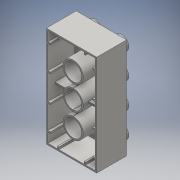
# Autodesk Inventor part: klarDupplo
Saved by Autodesk Inventor 2016 (Build 200138000, 138)
## iProperties
Created: 2017-02-13
Part Number: klarDupplo
Material: Generic
Document SubType Name: Modeling
Designer: 16wise
Density: 1 g/cm^3
Appearance: Default
Author: 16wise
Autodesk Inventor part; units mm, degrees
ref_plane "YZ Plane" through (0, 0, 0) normal (1, 0, 0) x (0, 1, 0)
ref_plane "XZ Plane" through (0, 0, 0) normal (0, 1, 0) x (-1, 0, 0)
ref_plane "XY Plane" through (0, 0, 0) normal (0, 0, 1) x (1, 0, 0)
sketch "Sketch1" plane through (0, 0, 0) normal (0, 1, 0) x (-1, 0, 0)
  line L0 (-16, 32) -> (16, 32)
  line L1 (16, 32) -> (16, -32)
  line L2 (16, -32) -> (-16, -32)
  line L3 (-16, -32) -> (-16, 32)
  line L4 (-16, 32) -> (16, -32) construction
  line L5 (16, 32) -> (-16, -32) construction
  point P0 (0, 0)
  dimension "d0" = 32
  dimension "d1" = 64
  constraints: 12 end point, 2 midpoint, 2 parallel, 1 horizontal, 1 perpendicular
  measures "d0" distance of L1.end L2.end
  measures "d1" distance of L0.end L1.end
extrude "Extrusion1" add sketch "Sketch1" along normal blind 19
sketch "Sketch2" plane through (0, 19, 0) normal (0, 1, 0) x (1, 0, 0)
  line L0 (-16, -32) -> (16, -32) projected
  line L1 (16, -32) -> (16, 32) projected
  line L2 (16, 32) -> (-16, 32) projected
  line L3 (-16, 32) -> (-16, -32) projected
  line L4 (-13, -29) -> (13, -29)
  line L5 (13, -29) -> (13, 29)
  line L6 (13, 29) -> (-13, 29)
  line L7 (-13, 29) -> (-13, -29)
  circle A0 centre (-8.5, -24.5) radius 4.5
  circle A1 centre (8.5, -24.5) radius 4.5
  line L8 (-16, 32) -> (-16, -32) projected
  circle A2 centre (-8.5, -8.2) radius 4.5
  circle A3 centre (-8.5, 8.1) radius 4.5
  circle A4 centre (-8.5, 24.4) radius 4.5
  circle A5 centre (8.5, -8.2) radius 4.5
  circle A6 centre (8.5, 8.1) radius 4.5
  circle A7 centre (8.5, 24.4) radius 4.5
  point P0 (0, 0)
  dimension "d4" = 3
  dimension "d5" = 9
  dimension "d6" = 9
  dimension "d9" = 16.3
  dimension "d16" = 16.3
  constraints: 8 centre point, 8 end point, 4 tangent, 2 vertical, 15 other
  measures "d4" distance between parallel lines of L3 L7
  measures "d5" diameter of A0
  measures "d6" diameter of A1
  measures "d9" distance of A0.centre A2.centre
  measures "d16" distance of A1.centre A5.centre
extrude "Extrusion2" add sketch "Sketch2" along normal blind 4.5 contours A5 | A6 | A7 | A4 | A3 | A2 | A0 | A1
sketch "Sketch3" plane through (-8.5, 23.5, 24.5) normal (0, 1, 0) x (1, 0, 0)
  circle A0 centre (0, 0) radius 3.5
  point P0 (8.5, 24.5)
  dimension "d23" = 7
  constraints: 1 centre point
  measures "d23" diameter of A0
extrude "Extrusion3" cut sketch "Sketch3" against normal blind 4.5
sketch "Sketch4" plane through (-8.5, 23.5, 8.2) normal (0, 1, 0) x (1, 0, 0)
  circle A0 centre (0, 0) radius 3.5
  point P0 (8.5, 8.2)
  dimension "d26" = 7
  constraints: 1 centre point
  measures "d26" diameter of A0
extrude "Extrusion4" cut sketch "Sketch4" against normal blind 4.5
sketch "Sketch5" plane through (-8.5, 23.5, -8.1) normal (0, 1, 0) x (1, 0, 0)
  circle A0 centre (0, 0) radius 3.5
  point P0 (8.5, -8.1)
  dimension "d29" = 7
  constraints: 1 centre point
  measures "d29" diameter of A0
extrude "Extrusion5" cut sketch "Sketch5" against normal blind 4.5
sketch "Sketch6" plane through (-8.5, 23.5, -24.4) normal (0, 1, 0) x (1, 0, 0)
  circle A0 centre (0, 0) radius 3.5
  point P0 (8.5, -24.4)
  dimension "d32" = 7
  constraints: 1 centre point
  measures "d32" diameter of A0
extrude "Extrusion6" cut sketch "Sketch6" against normal blind 4.5
sketch "Sketch7" plane through (8.5, 23.5, 24.5) normal (0, 1, 0) x (1, 0, 0)
  circle A0 centre (0, 0) radius 3.5
  point P0 (-8.5, 24.5)
  dimension "d35" = 7
  constraints: 1 centre point
  measures "d35" diameter of A0
extrude "Extrusion7" cut sketch "Sketch7" against normal blind 4.5
sketch "Sketch8" plane through (8.5, 23.5, 8.2) normal (0, 1, 0) x (1, 0, 0)
  circle A0 centre (0, 0) radius 4.5 projected
  circle A1 centre (0, 0) radius 3.5
  point P0 (-8.5, 8.2)
  dimension "d38" = 7
  constraints: 1 centre point, 1 coincident
  measures "d38" diameter of A1
extrude "Extrusion8" cut sketch "Sketch8" against normal blind 4.5 contours A1
sketch "Sketch9" plane through (8.5, 23.5, -8.1) normal (0, 1, 0) x (1, 0, 0)
  circle A0 centre (0, 0) radius 3.5
  point P0 (-8.5, -8.1)
  dimension "d41" = 7
  constraints: 1 centre point
  measures "d41" diameter of A0
extrude "Extrusion9" cut sketch "Sketch9" against normal blind 4.5
sketch "Sketch10" plane through (8.5, 23.5, -24.4) normal (0, 1, 0) x (1, 0, 0)
  circle A0 centre (0, 0) radius 3.5
  point P0 (-8.5, -24.4)
  dimension "d44" = 7
  constraints: 1 centre point
  measures "d44" diameter of A0
extrude "Extrusion10" cut sketch "Sketch10" against normal blind 4.5
sketch "Sketch11" plane through (0, 0, 0) normal (0, -1, 0) x (1, 0, 0)
  line L0 (16, 32) -> (-16, 32) projected
  line L1 (-16, 32) -> (-16, -32) projected
  line L2 (-16, -32) -> (16, -32) projected
  line L3 (16, -32) -> (16, 32) projected
  line L4 (15, -31) -> (-15, -31)
  line L5 (-15, -31) -> (-15, 31)
  line L6 (-15, 31) -> (15, 31)
  line L7 (15, 31) -> (15, -31)
  point P0 (0, 0)
  dimension "d47" = 1
  constraints: 8 end point, 3 other
  measures "d47" distance between parallel lines of L2 L4
extrude "Extrusion11" cut sketch "Sketch11" against normal blind 17 contours L4 L5 L6 L7
sketch "Sketch12" plane through (0, 17, 0) normal (0, -1, 0) x (1, 0, 0)
  circle A0 centre (0, 0) radius 6.5
  line L0 (15, -31) -> (-15, -31) projected
  line L1 (15, 31) -> (15, -31) projected
  line L2 (-15, 31) -> (15, 31) projected
  line L3 (-15, -31) -> (-15, 31) projected
  circle A1 centre (0, -15.5) radius 6.5
  circle A2 centre (0, 15.5) radius 6.5
  dimension "d50" = 13
  dimension "d53" = 15.5
  dimension "d60" = 15.5
  constraints: 3 centre point, 2 vertical, 1 coincident, 4 other
  measures "d50" diameter of A0
  measures "d53" distance of A0.centre A1.centre
  measures "d60" distance of A0.centre A2.centre
extrude "Extrusion12" add sketch "Sketch12" along normal blind 16 contours A0 | A1 | A2
sketch "Sketch13" plane through (0, 1, -15.5) normal (0, -1, 0) x (1, 0, 0)
  circle A0 centre (0, 0) radius 5.5
  circle A1 centre (0, 15.5) radius 5.5
  dimension "d67" = 11
  dimension "d68" = 11
  constraints: 2 centre point, 1 coincident
  measures "d67" diameter of A0
  measures "d68" diameter of A1
extrude "Extrusion13" cut sketch "Sketch13" against normal blind 16
sketch "Sketch14" plane through (0, 1, 15.5) normal (0, -1, 0) x (1, 0, 0)
  circle A0 centre (0, 0) radius 6.5 projected
  circle A1 centre (0, 0) radius 5.5
  point P0 (0, -15.5)
  dimension "d71" = 11
  constraints: 1 centre point, 1 coincident
  measures "d71" diameter of A1
extrude "Extrusion14" cut sketch "Sketch14" against normal blind 16 contours A1
sketch "Sketch15" plane through (0, 17, 0) normal (0, -1, 0) x (1, 0, 0)
  line L0 (-15, 0.5) -> (15, 0.5)
  line L1 (15, 0.5) -> (15, -0.5)
  line L2 (15, -0.5) -> (-15, -0.5)
  line L3 (-15, -0.5) -> (-15, 0.5)
  line L4 (-15, 0.5) -> (15, -0.5) construction
  line L5 (15, 0.5) -> (-15, -0.5) construction
  point P0 (0, 0)
  dimension "d74" = 30
  dimension "d75" = 1
  constraints: 12 end point, 2 midpoint, 2 parallel, 1 horizontal, 1 perpendicular
  measures "d74" distance of L1.end L2.end
  measures "d75" distance of L0.end L1.end
extrude "Extrusion15" add sketch "Sketch15" along normal blind 16
sketch "Sketch16" plane through (0, 1, 0) normal (0, -1, 0) x (1, 0, 0)
  arc A0 (5.4772, 0.5) -> (-5.4772, 0.5) centre (0, 0) ccw projected
  arc A1 (-5.4772, -0.5) -> (5.4772, -0.5) centre (0, 0) ccw projected
  line L0 (5.4772, 0.5) -> (5.4772, -0.5)
  line L1 (-5.4772, -0.5) -> (5.4772, -0.5) projected
  line L2 (-5.4772, 0.5) -> (-5.4772, -0.5)
  line L3 (-5.4772, -0.5) -> (5.4772, -0.5)
  line L4 (5.4772, 0.5) -> (-5.4772, 0.5) projected
  line L5 (5.4772, -0.5) -> (5.4772, 0.5)
  constraints: 8 end point, 2 vertical, 1 parallel, 1 perpendicular
extrude "Extrusion16" add sketch "Sketch16" against normal blind 16 contours L0 L1 L2 L4
sketch "Sketch17" plane through (0, 1, 0) normal (0, -1, 0) x (1, 0, 0)
  line L0 (5.4772, 0.5) -> (-5.4772, 0.5) projected
  line L1 (-5.4772, 0.5) -> (5.4772, 0.5)
  arc A0 (-5.4772, -0.5) -> (5.4772, -0.5) centre (0, 0) ccw projected
  arc A1 (5.4772, 0.5) -> (-5.4772, 0.5) centre (0, 0) ccw projected
  line L2 (5.4772, 0.5) -> (-5.4772, -0.5)
  line L3 (-5.4772, -0.5) -> (5.4772, -0.5) projected
  line L4 (-5.4772, -0.5) -> (-5.4772, 0.5)
  line L5 (5.4772, -0.5) -> (5.4772, 0.5)
  constraints: 8 end point, 2 equal length, 1 perpendicular
extrude "Extrusion17" cut sketch "Sketch17" against normal blind 16 contours L2 L4 L0 | L5 L3 L2
sketch "Sketch18" plane through (0, 17, 0) normal (0, -1, 0) x (1, 0, 0)
  circle A0 centre (0, 15.5) radius 6.5 projected
  line L0 (-0.25, -9.0048) -> (0.25, -9.0048)
  line L1 (0.25, -9.0048) -> (0.25, 9.0048)
  line L2 (0.25, 9.0048) -> (-0.25, 9.0048)
  line L3 (-0.25, 9.0048) -> (-0.25, -9.0048)
  line L4 (-0.25, -9.0048) -> (0.25, 9.0048) construction
  line L5 (0.25, -9.0048) -> (-0.25, 9.0048) construction
  point P0 (0, 0)
  dimension "d82" = 0.5
  constraints: 12 end point, 2 midpoint, 2 parallel, 1 horizontal, 1 perpendicular, 2 other
  measures "d82" distance of L2.end L1.end
extrude "Extrusion18" add sketch "Sketch18" along normal blind 16 contours L2 A0 | A0 L1 L0 L3 picked at (-0.0278, 9.0034)
sketch "Sketch19" plane through (0, 1, 0) normal (0, -1, 0) x (1, 0, 0)
  line L0 (0.25, 5.4943) -> (0.25, -5.4943) projected
  line L1 (-0.25, -5.4943) -> (0.25, -5.4943)
  line L2 (0.25, -5.4943) -> (0.25, 5.4943)
  line L3 (0.25, 5.4943) -> (-0.25, 5.4943)
  line L4 (-0.25, 5.4943) -> (-0.25, -5.4943)
  line L5 (-0.25, -5.4943) -> (0.25, 5.4943) construction
  line L6 (0.25, -5.4943) -> (-0.25, 5.4943) construction
  point P0 (0, 0)
  constraints: 12 end point, 2 midpoint, 2 parallel, 1 horizontal, 1 perpendicular
extrude "Extrusion19" cut sketch "Sketch19" against normal blind 16
sketch "Sketch20" plane through (0, 0, 0) normal (0, -1, 0) x (1, 0, 0)
  line L0 (15, -31) -> (-15, -31) projected
  line L1 (15, -31) -> (8, -31)
  line L2 (8, -31) -> (8, -24)
  line L3 (8, -24) -> (15, -24)
  line L4 (15, -24) -> (15, -31)
  point P0 (0, 0)
  dimension "d87" = 7
  dimension "d88" = 7
  constraints: 8 end point, 2 parallel, 1 horizontal, 1 perpendicular
  measures "d87" distance of L2.end L3.end
  measures "d88" distance of L1.end L2.end
extrude "Extrusion20" add sketch "Sketch20" against normal blind 16
sketch "Sketch21" plane through (0, 0, 0) normal (0, -1, 0) x (1, 0, 0)
  line L0 (15, -31) -> (-15, -31) projected
  line L1 (15, -31) -> (9, -31)
  line L2 (9, -31) -> (9, -25)
  line L3 (9, -25) -> (15, -25)
  line L4 (15, -25) -> (15, -31)
  point P0 (0, 0)
  dimension "d91" = 6
  dimension "d92" = 6
  constraints: 8 end point, 2 parallel, 1 horizontal, 1 perpendicular
  measures "d91" distance of L2.end L3.end
  measures "d92" distance of L1.end L2.end
extrude "Extrusion21" cut sketch "Sketch21" against normal blind 16
sketch "Sketch22" plane through (0, 1, 0) normal (0, -1, 0) x (1, 0, 0)
  line L0 (-0.25, 6.4952) -> (-0.25, 9.0048) projected
  line L1 (0.25, 9.0048) -> (0.25, 6.4952) projected
  line L2 (-0.25, 9.0048) -> (0.25, 9.0048)
  line L3 (0.25, 9.0048) -> (0.25, 6.4952)
  line L4 (0.25, 6.4952) -> (-0.25, 6.4952)
  line L5 (-0.25, 6.4952) -> (-0.25, 9.0048)
  point P0 (0, 0)
  constraints: 8 end point, 2 parallel, 1 horizontal, 1 perpendicular
extrude "Extrusion22" cut sketch "Sketch22" against normal blind 2.5
sketch "Sketch23" plane through (0, 1, 0) normal (0, -1, 0) x (1, 0, 0)
  arc A0 (-6.4807, -0.5) -> (-0.25, -6.4952) centre (0, 0) ccw projected
  arc A1 (-0.25, -9.0048) -> (0.25, -9.0048) centre (0, -15.5) ccw projected
  line L0 (-0.25, -6.4952) -> (0.25, -6.4952)
  line L1 (0.25, -6.4952) -> (0.25, -9.0048)
  line L2 (0.25, -9.0048) -> (-0.25, -9.0048)
  line L3 (-0.25, -9.0048) -> (-0.25, -6.4952)
  constraints: 8 end point, 2 parallel, 1 horizontal, 1 perpendicular
extrude "Extrusion23" cut sketch "Sketch23" against normal blind 2.5 contours L3 L0 L1 L2
sketch "Sketch24" plane through (0, 1, 0) normal (0, -1, 0) x (1, 0, 0)
  line L0 (-6.4807, 0.5) -> (-15, 0.5) projected
  line L1 (-15, -0.5) -> (-6.4807, -0.5) projected
  line L2 (-15, 0.5) -> (-6.4807, 0.5)
  line L3 (-6.4807, 0.5) -> (-6.4807, -0.5)
  line L4 (-6.4807, -0.5) -> (-15, -0.5)
  line L5 (-15, -0.5) -> (-15, 0.5)
  point P0 (0, 0)
  constraints: 8 end point, 2 parallel, 1 horizontal, 1 perpendicular
extrude "Extrusion24" cut sketch "Sketch24" against normal blind 3.5
sketch "Sketch25" plane through (0, 1, 0) normal (0, -1, 0) x (1, 0, 0)
  line L0 (15, 0.5) -> (6.4807, 0.5) projected
  line L1 (6.4807, -0.5) -> (15, -0.5) projected
  line L2 (6.4807, 0.5) -> (15, 0.5)
  line L3 (15, 0.5) -> (15, -0.5)
  line L4 (15, -0.5) -> (6.4807, -0.5)
  line L5 (6.4807, -0.5) -> (6.4807, 0.5)
  point P0 (0, 0)
  constraints: 8 end point, 2 parallel, 1 horizontal, 1 perpendicular
extrude "Extrusion25" cut sketch "Sketch25" against normal blind 3.5
sketch "Sketch26" plane through (0, 0, 0) normal (0, -1, 0) x (1, 0, 0)
  line L0 (-15, 31) -> (15, 31) projected
  line L1 (15, 31) -> (8, 31)
  line L2 (8, 31) -> (8, 24)
  line L3 (8, 24) -> (15, 24)
  line L4 (15, 24) -> (15, 31)
  point P0 (0, 0)
  dimension "d103" = 7
  dimension "d104" = 7
  constraints: 8 end point, 2 parallel, 1 horizontal, 1 perpendicular
  measures "d103" distance of L3.end L2.end
  measures "d104" distance of L2.end L1.end
extrude "Extrusion26" add sketch "Sketch26" against normal blind 18
sketch "Sketch27" plane through (0, 0, 0) normal (0, -1, 0) x (1, 0, 0)
  line L0 (-15, 0.5) -> (-15, 31) projected
  line L1 (-15, 31) -> (-8, 31)
  line L2 (-8, 31) -> (-8, 24)
  line L3 (-8, 24) -> (-15, 24)
  line L4 (-15, 24) -> (-15, 31)
  point P0 (0, 0)
  dimension "d107" = 7
  dimension "d108" = 7
  constraints: 8 end point, 2 parallel, 1 horizontal, 1 perpendicular
  measures "d107" distance of L2.end L3.end
  measures "d108" distance of L1.end L2.end
extrude "Extrusion27" add sketch "Sketch27" against normal blind 18
sketch "Sketch28" plane through (0, 0, 0) normal (0, -1, 0) x (1, 0, 0)
  line L0 (-15, -31) -> (-15, -0.5) projected
  line L1 (-15, -31) -> (-8, -31)
  line L2 (-8, -31) -> (-8, -24)
  line L3 (-8, -24) -> (-15, -24)
  line L4 (-15, -24) -> (-15, -31)
  point P0 (0, 0)
  dimension "d111" = 7
  dimension "d112" = 7
  constraints: 8 end point, 2 parallel, 1 horizontal, 1 perpendicular
  measures "d111" distance of L3.end L2.end
  measures "d112" distance of L2.end L1.end
extrude "Extrusion28" add sketch "Sketch28" against normal blind 18
sketch "Sketch29" plane through (0, 0, 0) normal (0, -1, 0) x (1, 0, 0)
  line L0 (15, 31) -> (9, 31)
  line L1 (9, 31) -> (9, 25)
  line L2 (9, 25) -> (15, 25)
  line L3 (15, 25) -> (15, 31)
  line L4 (-15, 31) -> (-9, 31)
  line L5 (-9, 31) -> (-9, 25)
  line L6 (-9, 25) -> (-15, 25)
  line L7 (-15, 25) -> (-15, 31)
  line L8 (-15, -31) -> (-9, -31)
  line L9 (-9, -31) -> (-9, -25)
  line L10 (-9, -25) -> (-15, -25)
  line L11 (-15, -25) -> (-15, -31)
  point P0 (0, 0)
  dimension "d115" = 6
  dimension "d116" = 6
  dimension "d117" = 6
  dimension "d118" = 6
  dimension "d119" = 6
  constraints: 24 end point, 6 parallel, 3 horizontal, 3 perpendicular, 3 point on line
  measures "d115" distance of L2.end L1.end
  measures "d116" distance of L1.end L0.end
  measures "d117" distance of L5.end L6.end
  measures "d118" distance of L10.end L9.end
  measures "d119" distance of L9.end L8.end
extrude "Extrusion29" cut sketch "Sketch29" against normal blind 18
sketch "Sketch30" plane through (0, 0, 0) normal (0, -1, 0) x (1, 0, 0)
  line L0 (-8, -24) -> (-15, -24) projected
  line L1 (-15, -25) -> (-9, -25) projected
  line L2 (-8, -24) -> (-13.5, -24)
  line L3 (-13.5, -24) -> (-13.5, -25)
  line L4 (-13.5, -25) -> (-8, -25)
  line L5 (-8, -25) -> (-8, -24)
  point P0 (0, 0)
  dimension "d122" = 5.5
  constraints: 8 end point, 2 parallel, 1 horizontal, 1 perpendicular, 1 point on line
  measures "d122" distance of L4.end L3.end
extrude "Extrusion30" cut sketch "Sketch30" against normal blind 17
sketch "Sketch31" plane through (0, 0, 0) normal (0, -1, 0) x (1, 0, 0)
  line L0 (-9, -25) -> (-13.5, -25) projected
  line L1 (-9, -25) -> (-8, -25)
  line L2 (-8, -25) -> (-8, -29.5)
  line L3 (-8, -29.5) -> (-9, -29.5)
  line L4 (-9, -29.5) -> (-9, -25)
  point P0 (0, 0)
  dimension "d125" = 1
  dimension "d126" = 4.5
  constraints: 8 end point, 2 parallel, 1 horizontal, 1 perpendicular
  measures "d125" distance of L2.end L3.end
  measures "d126" distance of L1.end L2.end
extrude "Extrusion31" cut sketch "Sketch31" against normal blind 17
sketch "Sketch32" plane through (0, 0, 0) normal (0, -1, 0) x (1, 0, 0)
  line L0 (8, -24) -> (15, -24) projected
  line L1 (9, -25) -> (15, -25) projected
  line L2 (8, -24) -> (13.5, -24)
  line L3 (13.5, -24) -> (13.5, -25)
  line L4 (13.5, -25) -> (8, -25)
  line L5 (8, -25) -> (8, -24)
  point P0 (0, 0)
  dimension "d129" = 5.5
  constraints: 8 end point, 2 parallel, 1 horizontal, 1 perpendicular, 1 point on line
  measures "d129" distance of L3.end L4.end
extrude "Extrusion32" cut sketch "Sketch32" against normal blind 17
sketch "Sketch33" plane through (0, 0, 0) normal (0, -1, 0) x (1, 0, 0)
  line L0 (8, -25) -> (9, -25)
  line L1 (9, -25) -> (9, -29.5)
  line L2 (9, -29.5) -> (8, -29.5)
  line L3 (8, -29.5) -> (8, -25)
  point P0 (0, 0)
  dimension "d132" = 1
  dimension "d133" = 4.5
  constraints: 8 end point, 2 parallel, 1 horizontal, 1 perpendicular
  measures "d132" distance of L1.end L2.end
  measures "d133" distance of L0.end L1.end
extrude "Extrusion33" cut sketch "Sketch33" against normal blind 17
sketch "Sketch34" plane through (0, 0, 0) normal (0, -1, 0) x (1, 0, 0)
  line L0 (8, 24) -> (15, 24) projected
  line L1 (8, 24) -> (9, 24)
  line L2 (9, 24) -> (9, 29.5)
  line L3 (9, 29.5) -> (8, 29.5)
  line L4 (8, 29.5) -> (8, 24)
  point P0 (0, 0)
  dimension "d136" = 1
  dimension "d137" = 5.5
  constraints: 8 end point, 2 parallel, 1 horizontal, 1 perpendicular
  measures "d136" distance of L3.end L2.end
  measures "d137" distance of L2.end L1.end
extrude "Extrusion34" cut sketch "Sketch34" against normal blind 17
sketch "Sketch35" plane through (0, 0, 0) normal (0, -1, 0) x (1, 0, 0)
  line L0 (15, 25) -> (9, 25) projected
  line L1 (15, 24) -> (9, 24) projected
  line L2 (9, 25) -> (13.5, 25)
  line L3 (13.5, 25) -> (13.5, 24)
  line L4 (13.5, 24) -> (9, 24)
  line L5 (9, 24) -> (9, 25)
  point P0 (0, 0)
  dimension "d140" = 4.5
  constraints: 8 end point, 2 parallel, 1 horizontal, 1 perpendicular, 1 point on line
  measures "d140" distance of L3.end L4.end
extrude "Extrusion35" cut sketch "Sketch35" against normal blind 17
sketch "Sketch36" plane through (0, 0, 0) normal (0, -1, 0) x (1, 0, 0)
  line L0 (-8, 31) -> (-8, 24) projected
  line L1 (-8, 24) -> (-9, 24)
  line L2 (-9, 24) -> (-9, 29.5)
  line L3 (-9, 29.5) -> (-8, 29.5)
  line L4 (-8, 29.5) -> (-8, 24)
  point P0 (0, 0)
  dimension "d143" = 1
  dimension "d144" = 5.5
  constraints: 8 end point, 2 parallel, 1 horizontal, 1 perpendicular
  measures "d143" distance of L2.end L3.end
  measures "d144" distance of L1.end L2.end
extrude "Extrusion36" cut sketch "Sketch36" against normal blind 17
sketch "Sketch37" plane through (0, 0, 0) normal (0, -1, 0) x (1, 0, 0)
  line L0 (-9, 25) -> (-9, 29.5) projected
  line L1 (-9, 24) -> (-15, 24) projected
  line L2 (-9, 25) -> (-13.5, 25)
  line L3 (-13.5, 25) -> (-13.5, 24)
  line L4 (-13.5, 24) -> (-9, 24)
  line L5 (-9, 24) -> (-9, 25)
  point P0 (0, 0)
  dimension "d147" = 4.5
  constraints: 8 end point, 2 parallel, 1 horizontal, 1 perpendicular, 1 point on line
  measures "d147" distance of L4.end L3.end
extrude "Extrusion37" cut sketch "Sketch37" against normal blind 17
sketch "Sketch40" plane through (0, 18, 0) normal (0, -1, 0) x (1, 0, 0)
  line L0 (-9, 31) -> (-9, 25) projected
  line L1 (-15, 31) -> (-9, 31) projected
  line L2 (-9, 25) -> (-15, 25)
  line L3 (-15, 25) -> (-15, 31)
  line L4 (-15, 31) -> (-9, 31)
  line L5 (-9, 31) -> (-9, 25)
  point P0 (0, 0)
  constraints: 8 end point, 2 parallel, 1 horizontal, 1 perpendicular
extrude "Extrusion38" add sketch "Sketch40" along normal blind 1
sketch "Sketch41" plane through (0, 18, 0) normal (0, -1, 0) x (1, 0, 0)
  line L0 (9, 29.5) -> (9, 25) projected
  line L1 (9, 31) -> (15, 31) projected
  line L2 (9, 25) -> (15, 25)
  line L3 (15, 25) -> (15, 31)
  line L4 (15, 31) -> (9, 31)
  line L5 (9, 31) -> (9, 25)
  point P0 (0, 0)
  constraints: 8 end point, 2 parallel, 1 horizontal, 1 perpendicular
extrude "Extrusion39" add sketch "Sketch41" along normal blind 1
sketch "Sketch42" plane through (0, 18, 0) normal (0, -1, 0) x (1, 0, 0)
  line L0 (-15, -25) -> (-9, -25) projected
  line L1 (-15, -31) -> (-15, -25) projected
  line L2 (-9, -25) -> (-15, -25)
  line L3 (-15, -25) -> (-15, -31)
  line L4 (-15, -31) -> (-9, -31)
  line L5 (-9, -31) -> (-9, -25)
  point P0 (0, 0)
  constraints: 8 end point, 2 parallel, 1 horizontal, 1 perpendicular
extrude "Extrusion40" add sketch "Sketch42" along normal blind 1
sketch "Sketch43" plane through (0, 1, 0) normal (0, -1, 0) x (1, 0, 0)
  line L0 (9, 31) -> (15, 31) projected
  line L1 (15, 31) -> (15, 8)
  line L2 (15, 24) -> (15, 0.5) projected
  line L3 (15, 8) -> (13.5, 8)
  line L4 (13.5, 8) -> (13.5, 7)
  line L5 (13.5, 7) -> (15, 7)
  line L6 (15, 7) -> (15, 8)
  line L7 (-15, 31) -> (-9, 31) projected
  line L8 (-15, 31) -> (-15, 9)
  line L9 (-15, 0.5) -> (-15, 24) projected
  line L10 (-15, 9) -> (-13.5, 9)
  line L11 (-13.5, 9) -> (-13.5, 8)
  line L12 (-13.5, 8) -> (-15, 8)
  line L13 (-15, 8) -> (-15, 9)
  line L14 (15, -0.5) -> (15, -31) projected
  line L15 (15, -31) -> (15, -9)
  line L16 (15, -9) -> (13.5, -9)
  line L17 (13.5, -9) -> (13.5, -8)
  line L18 (13.5, -8) -> (15, -8)
  line L19 (15, -8) -> (15, -9)
  line L20 (-15, -31) -> (-15, -25) projected
  line L21 (-15, -31) -> (-15, -9)
  line L22 (-15, -24) -> (-15, -0.5) projected
  line L23 (-15, -9) -> (-13.5, -9)
  line L24 (-13.5, -9) -> (-13.5, -8)
  line L25 (-13.5, -8) -> (-15, -8)
  line L26 (-15, -8) -> (-15, -9)
  point P0 (0, 0)
  dimension "d156" = 23
  dimension "d157" = 1.5
  dimension "d158" = 1
  dimension "d159" = 22
  dimension "d160" = 1.5
  dimension "d161" = 1
  dimension "d162" = 22
  dimension "d163" = 1.5
  dimension "d164" = 1
  dimension "d165" = 1.5
  dimension "d166" = 1
  constraints: 40 end point, 8 parallel, 4 horizontal, 4 perpendicular, 4 point on line
  measures "d156" distance of L0.end L1.end
  measures "d157" distance of L5.end L4.end
  measures "d158" distance of L4.end L3.end
  measures "d159" distance of L7.start L8.end
  measures "d160" distance of L11.end L12.end
  measures "d161" distance of L10.end L11.end
  measures "d162" distance of L14.end L15.end
  measures "d163" distance of L17.end L18.end
  measures "d164" distance of L16.end L17.end
  measures "d165" distance of L25.end L24.end
  measures "d166" distance of L24.end L23.end
extrude "Extrusion41" add sketch "Sketch43" against normal blind 18
sketch "Sketch44" plane through (0, 1, 0) normal (0, -1, 0) x (1, 0, 0)
  line L0 (13.5, 7) -> (15, 7) projected
  line L1 (13.5, 8) -> (15, 8)
  line L2 (15, 8) -> (15, 7)
  line L3 (15, 7) -> (13.5, 7)
  line L4 (13.5, 7) -> (13.5, 8)
  line L5 (15, -9) -> (13.5, -9) projected
  line L6 (13.5, -9) -> (15, -9)
  line L7 (15, -9) -> (15, -8)
  line L8 (15, -8) -> (13.5, -8)
  line L9 (13.5, -8) -> (13.5, -9)
  line L10 (-13.5, -9) -> (-15, -9) projected
  line L11 (-15, -8) -> (-13.5, -8)
  line L12 (-13.5, -8) -> (-13.5, -9)
  line L13 (-13.5, -9) -> (-15, -9)
  line L14 (-15, -9) -> (-15, -8)
  line L15 (-13.5, 8) -> (-15, 8)
  line L16 (-15, 8) -> (-15, 9)
  line L17 (-15, 9) -> (-13.5, 9)
  line L18 (-13.5, 9) -> (-13.5, 8)
  point P0 (0, 0)
  dimension "d169" = 1.5
  dimension "d170" = 1
  dimension "d171" = 1.5
  dimension "d172" = 1
  constraints: 32 end point, 8 parallel, 4 horizontal, 4 perpendicular, 3 point on line
  measures "d169" distance of L8.end L7.end
  measures "d170" distance of L7.end L6.end
  measures "d171" distance of L16.end L17.end
  measures "d172" distance of L15.end L16.end
extrude "Extrusion42" add sketch "Sketch44" along normal blind 1
sketch "Sketch45" plane through (0, 17, 0) normal (0, -1, 0) x (1, 0, 0)
  point P0 (0, 0)
body "Solid1"
